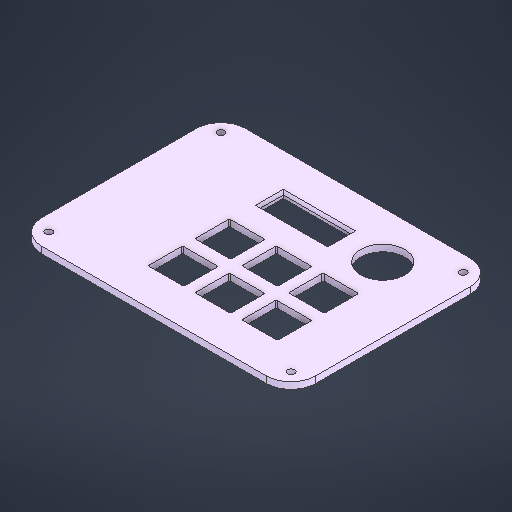
# Autodesk Inventor part: Middle
Saved by Autodesk Inventor 2026.2 (Build 302298000, 298)
## iProperties
Created: 2026-02-15
Part Number: Middle
Material: Generic
Document SubType Name: Modeling
Designer: bh
Density: 1 g/cm^3
Appearance: Default
Author: bh
Autodesk Inventor part; units mm, degrees
ref_plane "YZ Plane" through (0, 0, 0) normal (1, 0, 0) x (0, 1, 0)
ref_plane "XZ Plane" through (0, 0, 0) normal (0, 1, 0) x (-1, 0, 0)
ref_plane "XY Plane" through (0, 0, 0) normal (0, 0, 1) x (1, 0, 0)
sketch "Sketch1" plane through (0, 0, 0) normal (0, 1, 0) x (-1, 0, 0)
  line L0 (-27.2265, 26.5665) -> (-13.7265, 26.5665)
  line L1 (-27.2265, 12.5665) -> (-13.7265, 12.5665)
  line L2 (-27.7265, 26.0665) -> (-27.7265, 13.0665)
  line L3 (-13.2265, 26.0665) -> (-13.2265, 13.0665)
  arc A0 (-27.2265, 26.5665) -> (-27.7265, 26.0665) centre (-27.2265, 26.0665) ccw
  arc A1 (-13.2265, 26.0665) -> (-13.7265, 26.5665) centre (-13.7265, 26.0665) ccw
  arc A2 (-27.7265, 13.0665) -> (-27.2265, 12.5665) centre (-27.2265, 13.0665) ccw
  arc A3 (-13.7265, 12.5665) -> (-13.2265, 13.0665) centre (-13.7265, 13.0665) ccw
  line L4 (-8.1765, 26.5665) -> (4.8235, 26.5665)
  line L5 (-8.1765, 12.5665) -> (4.8235, 12.5665)
  line L6 (-8.6765, 26.0665) -> (-8.6765, 13.0665)
  arc A4 (-8.1765, 26.5665) -> (-8.6765, 26.0665) centre (-8.1765, 26.0665) ccw
  arc A5 (-8.6765, 13.0665) -> (-8.1765, 12.5665) centre (-8.1765, 13.0665) ccw
  line L7 (10.8735, 26.5665) -> (23.8735, 26.5665)
  line L8 (10.8735, 12.5665) -> (23.8735, 12.5665)
  line L9 (10.3735, 26.0665) -> (10.3735, 13.0665)
  arc A6 (10.8735, 26.5665) -> (10.3735, 26.0665) centre (10.8735, 26.0665) ccw
  arc A7 (10.3735, 13.0665) -> (10.8735, 12.5665) centre (10.8735, 13.0665) ccw
  line L10 (-28.6565, 28.2795) -> (28.4935, 28.2795)
  line L11 (-28.6565, -9.8205) -> (-28.6565, 28.2795)
  line L12 (28.4935, -9.8205) -> (28.4935, 28.2795)
  line L13 (-28.6565, 28.2795) -> (-37.9765, 28.2795)
  line L14 (-37.9765, 28.2795) -> (-37.9765, 31.2995)
  line L15 (-37.9765, 31.2995) -> (-28.6565, 31.2995)
  line L16 (-28.6565, 31.2995) -> (-28.6565, 28.2795)
  line L17 (-37.9765, 31.2995) -> (53.4235, 31.2995)
  line L18 (53.4235, 31.2995) -> (53.4235, -31.6005)
  line L19 (53.4235, -31.6005) -> (-37.9765, -31.6005)
  line L20 (-37.9765, -31.6005) -> (-37.9765, 31.2995)
  line L21 (-37.9765, -31.6005) -> (-34.6365, -31.6005)
  line L22 (-37.9765, -20.5605) -> (-37.9765, -31.6005)
  line L23 (-17.165, -31.6005) -> (-34.6365, -31.6005)
  line L24 (-37.9765, -31.6005) -> (-26.9365, -31.6005)
  line L25 (-37.9765, -16.1605) -> (-37.9765, -31.6005)
  line L26 (-14.9265, -31.6005) -> (-26.9365, -31.6005)
  line L27 (-26.9365, -31.6005) -> (-14.9265, -31.6005)
  line L28 (53.4235, -31.6005) -> (-12.9716, -31.6005)
  line L29 (53.4235, -26.4105) -> (53.4235, -31.6005)
  line L30 (-37.9765, -31.6005) -> (-2.8865, -31.6005)
  line L31 (-37.9765, -9.8205) -> (-37.9765, -31.6005)
  line L32 (63.4235, -41.6005) -> (63.4235, 41.2995)
  line L33 (63.4235, 41.2995) -> (-47.9765, 41.2995)
  line L34 (63.4235, -41.6005) -> (-47.9765, -41.6005)
  line L35 (-47.9765, -41.6005) -> (-47.9765, 41.2995)
  line L36 (-37.9008, -41.6005) -> (53.4992, -41.6005)
  line L37 (-20.9315, -41.6005) -> (-34.0815, -41.6005)
  line L38 (-47.9008, -28.4505) -> (-68.6108, -28.4505) construction
  line L39 (-37.9765, -41.6005) -> (53.4235, -41.6005)
  line L40 (-21.0072, -41.6005) -> (-34.1572, -41.6005)
  line L41 (-48.2513, 31.2983) -> (-47.9765, -31.6005)
  line L42 (-47.9903, -28.4505) -> (-68.3765, -28.4505) construction
  line L43 (-47.9765, -31.6005) -> (-37.9765, -31.6005)
  line L44 (-37.9765, -31.6005) -> (-37.9765, -41.6005)
  line L45 (-37.9765, -41.6005) -> (-47.9765, -41.6005)
  line L46 (-47.9765, -41.6005) -> (-47.9765, -31.6005)
  line L47 (-47.9765, -41.6005) -> (-27.5765, -41.6005)
  line L48 (-27.5765, -41.6005) -> (-27.5765, -9.8205)
  line L49 (-27.5765, -9.8205) -> (-47.9765, -9.8205)
  line L50 (-47.9765, -9.8205) -> (-47.9765, -41.6005)
  line L51 (-47.9765, -41.6005) -> (-15.5765, -41.6005)
  line L52 (-15.5765, -41.6005) -> (-15.5765, -9.8205)
  line L53 (-15.5765, -9.8205) -> (-47.9765, -9.8205)
  line L54 (-47.9765, -9.8205) -> (-47.9765, -41.6005)
  line L55 (-47.9765, -41.6005) -> (-9.3811, -41.6005)
  line L56 (-9.3811, -41.6005) -> (-9.3811, -28.4505)
  line L57 (-9.3811, -28.4505) -> (-47.9765, -28.4505)
  line L58 (-47.9765, -28.4505) -> (-47.9765, -41.6005)
  line L59 (-27.5765, -28.4505) -> (-15.5765, -28.4505)
  line L60 (-15.5765, -28.4505) -> (-15.5765, -16.3505)
  line L61 (-15.5765, -16.3505) -> (-27.5765, -16.3505)
  line L62 (-27.5765, -16.3505) -> (-27.5765, -28.4505)
  line L63 (-21.5765, -28.4505) -> (-21.5765, -22.4005)
  line L64 (-21.5765, -22.4005) -> (-27.5765, -22.4005)
  circle A8 centre (-21.5765, -22.4005) radius 9
  line L65 (27.5574, -41.6005) -> (-5.1303, -41.6005)
  line L66 (-5.1303, -41.6005) -> (-5.1303, -17.8005)
  line L67 (-5.1303, -17.8005) -> (27.5574, -17.8005)
  line L68 (27.5574, -17.8005) -> (27.5574, -41.6005)
  line L69 (53.4235, -22.9498) -> (23.0635, -22.9498)
  line L70 (23.0635, -22.9498) -> (-3.5365, -22.9498)
  line L71 (23.0635, -17.8005) -> (23.0635, -26.6005)
  line L72 (23.0635, -26.6005) -> (-3.7865, -26.6005)
  line L73 (-3.7865, -26.6005) -> (-3.7865, -17.8005)
  line L74 (-3.7865, -17.8005) -> (23.0635, -17.8005)
  line L75 (23.0635, -17.8005) -> (23.0635, -26.6005)
  line L76 (-4.0365, -26.8505) -> (23.3135, -26.8505)
  line L77 (23.3135, -26.8505) -> (23.3135, -17.5505)
  line L78 (23.3135, -17.5505) -> (-4.0365, -17.5505)
  line L79 (-4.0365, -17.5505) -> (-4.0365, -26.8505)
  line L80 (-48.1765, 14.1732) -> (-27.9265, 14.1732)
  line L81 (-27.7265, 13.0665) -> (-27.7265, 13.0665)
  line L82 (-20.7265, 12.5665) -> (-20.7265, 12.5665)
  line L83 (-20.7265, 12.5665) -> (-20.7265, 12.5665)
  line L84 (-27.7265, 13.0665) -> (-27.7265, 13.0665)
  line L85 (-27.7265, 19.5665) -> (-13.2265, 19.5665)
  line L86 (-13.2265, 13.0665) -> (-13.2265, 13.0665)
  line L87 (-8.1765, 12.5665) -> (5.3235, 12.5665)
  arc A9 (-8.6765, 13.0665) -> (-8.1765, 12.5665) centre (-8.1765, 13.0665) ccw
  arc A10 (5.3235, 12.5665) -> (5.8235, 13.0665) centre (5.3235, 13.0665) ccw
  line L88 (-8.6765, 26.0665) -> (-8.6765, 13.0665)
  line L89 (5.8235, 26.0665) -> (5.8235, 13.0665)
  line L90 (-8.1765, 26.5665) -> (5.3235, 26.5665)
  arc A11 (-8.1765, 26.5665) -> (-8.6765, 26.0665) centre (-8.1765, 26.0665) ccw
  arc A12 (5.8235, 26.0665) -> (5.3235, 26.5665) centre (5.3235, 26.0665) ccw
  line L91 (10.8735, 12.5665) -> (24.3735, 12.5665)
  arc A13 (10.3735, 13.0665) -> (10.8735, 12.5665) centre (10.8735, 13.0665) ccw
  arc A14 (24.3735, 12.5665) -> (24.8735, 13.0665) centre (24.3735, 13.0665) ccw
  line L92 (10.3735, 26.0665) -> (10.3735, 13.0665)
  line L93 (24.8735, 26.0665) -> (24.8735, 13.0665)
  line L94 (10.8735, 26.5665) -> (24.3735, 26.5665)
  arc A15 (10.8735, 26.5665) -> (10.3735, 26.0665) centre (10.8735, 26.0665) ccw
  arc A16 (24.8735, 26.0665) -> (24.3735, 26.5665) centre (24.3735, 26.0665) ccw
  line L95 (17.3735, 12.5665) -> (17.3735, 12.5665)
  line L96 (17.3735, 12.5665) -> (17.3735, 12.5665)
  line L97 (24.8735, 13.0665) -> (24.8735, 13.0665)
  line L98 (-28.6565, 7.0165) -> (-28.6565, 9.2295)
  line L99 (-28.6565, 9.2295) -> (-27.2265, 9.2295)
  line L100 (-27.2265, -6.4831) -> (-13.7265, -6.4831)
  arc A17 (-27.7265, -5.9831) -> (-27.2265, -6.4831) centre (-27.2265, -5.9831) ccw
  arc A18 (-13.7265, -6.4831) -> (-13.2265, -5.9831) centre (-13.7265, -5.9831) ccw
  line L101 (-27.7265, 7.0169) -> (-27.7265, -5.9831)
  line L102 (-13.2265, 7.0169) -> (-13.2265, -5.9831)
  line L103 (-27.2265, 7.5169) -> (-13.7265, 7.5169)
  arc A19 (-27.2265, 7.5169) -> (-27.7265, 7.0169) centre (-27.2265, 7.0169) ccw
  arc A20 (-13.2265, 7.0169) -> (-13.7265, 7.5169) centre (-13.7265, 7.0169) ccw
  line L104 (-8.6765, 7.0169) -> (-8.6765, -5.9831)
  arc A21 (-8.1765, 7.5169) -> (-8.6765, 7.0169) centre (-8.1765, 7.0169) ccw
  line L105 (-8.1765, -6.4831) -> (4.8235, -6.4831)
  arc A22 (-8.6765, -5.9831) -> (-8.1765, -6.4831) centre (-8.1765, -5.9831) ccw
  line L106 (-8.1765, 7.5169) -> (4.8235, 7.5169)
  line L107 (10.3735, 7.0169) -> (10.3735, -5.9831)
  line L108 (10.8735, 7.5169) -> (23.8735, 7.5169)
  arc A23 (10.8735, 7.5169) -> (10.3735, 7.0169) centre (10.8735, 7.0169) ccw
  line L109 (10.8735, -6.4831) -> (23.8735, -6.4831)
  arc A24 (10.3735, -5.9831) -> (10.8735, -6.4831) centre (10.8735, -5.9831) ccw
  line L110 (-27.7265, -5.9831) -> (-27.7265, -5.9831)
  line L111 (-20.7265, -6.4831) -> (-20.7265, -6.4831)
  line L112 (-20.7265, -6.4831) -> (-20.7265, -6.4831)
  line L113 (-27.7265, -5.9831) -> (-27.7265, -5.9831)
  line L114 (-13.2265, -5.9831) -> (-13.2265, -5.9831)
  line L115 (-8.6765, 7.0169) -> (-8.6765, -5.9831)
  arc A25 (-8.1765, 7.5169) -> (-8.6765, 7.0169) centre (-8.1765, 7.0169) ccw
  line L116 (5.8235, 7.0169) -> (5.8235, -5.9831)
  line L117 (-8.1765, 7.5169) -> (5.3235, 7.5169)
  arc A26 (5.8235, 7.0169) -> (5.3235, 7.5169) centre (5.3235, 7.0169) ccw
  line L118 (-8.1765, -6.4831) -> (5.3235, -6.4831)
  arc A27 (5.3235, -6.4831) -> (5.8235, -5.9831) centre (5.3235, -5.9831) ccw
  arc A28 (-8.6765, -5.9831) -> (-8.1765, -6.4831) centre (-8.1765, -5.9831) ccw
  arc A29 (10.3735, -5.9831) -> (10.8735, -6.4831) centre (10.8735, -5.9831) ccw
  line L119 (10.8735, -6.4831) -> (24.3735, -6.4831)
  arc A30 (24.3735, -6.4831) -> (24.8735, -5.9831) centre (24.3735, -5.9831) ccw
  arc A31 (24.8735, 7.0169) -> (24.3735, 7.5169) centre (24.3735, 7.0169) ccw
  line L120 (24.8735, 7.0169) -> (24.8735, -5.9831)
  line L121 (10.8735, 7.5169) -> (24.3735, 7.5169)
  arc A32 (10.8735, 7.5169) -> (10.3735, 7.0169) centre (10.8735, 7.0169) ccw
  line L122 (17.3735, -6.4831) -> (17.3735, -6.4831)
  line L123 (17.3735, -6.4831) -> (17.3735, -6.4831)
  line L124 (24.8735, -5.9831) -> (24.8735, -5.9831)
  line L125 (10.3735, 7.0169) -> (10.3735, -5.9831)
  line L126 (-27.7265, 7.0169) -> (-27.7265, -5.9831)
  arc A33 (-27.2265, 7.5169) -> (-27.7265, 7.0169) centre (-27.2265, 7.0169) ccw
  line L127 (-27.2265, -6.4831) -> (-14.2265, -6.4831)
  arc A34 (-27.7265, -5.9831) -> (-27.2265, -6.4831) centre (-27.2265, -5.9831) ccw
  line L128 (-27.2265, 7.5169) -> (-14.2265, 7.5169)
  line L129 (-27.7265, 7.0169) -> (-27.7265, -5.9831)
  arc A35 (-27.2265, 7.5169) -> (-27.7265, 7.0169) centre (-27.2265, 7.0169) ccw
  line L130 (-13.2265, 7.0169) -> (-13.2265, -5.9831)
  line L131 (-27.2265, 7.5169) -> (-13.7265, 7.5169)
  arc A36 (-13.2265, 7.0169) -> (-13.7265, 7.5169) centre (-13.7265, 7.0169) ccw
  line L132 (-27.2265, -6.4831) -> (-13.7265, -6.4831)
  arc A37 (-13.7265, -6.4831) -> (-13.2265, -5.9831) centre (-13.7265, -5.9831) ccw
  arc A38 (-27.7265, -5.9831) -> (-27.2265, -6.4831) centre (-27.2265, -5.9831) ccw
  point P0 (10.8735, 26.5665)
  point P1 (10.8735, 12.5665)
  point P2 (10.3735, 13.0665)
  point P3 (-8.1765, 12.5665)
  point P4 (-8.6765, 13.0665)
  point P5 (-8.6765, 26.0665)
  point P6 (-14.2265, 26.5665)
  point P7 (-13.2265, 13.0665)
  point P8 (-14.2265, 12.5665)
  point P9 (-2.8865, -17.0492)
  point P10 (-6.5815, -26.4105)
  point P11 (23.7135, -17.6392)
  point P12 (23.3135, -17.8005)
  point P13 (-4.0365, -17.8005)
  point P14 (-1.6765, 12.5665)
  point P15 (-8.6765, 19.5665)
  point P16 (-8.6765, 0.5169)
  point P17 (-1.6765, -6.4831)
  point P18 (-8.1765, 7.5169)
  point P19 (-27.2265, 7.5169)
  point P20 (24.8735, 7.0169)
  point P21 (10.8735, 7.5169)
  point P22 (24.8735, 13.0665)
  point P23 (24.8735, 26.0665)
  point P24 (-20.7265, -6.4831)
  dimension "d8" = 9.32
  dimension "d9" = 3.02
  dimension "d11" = 62.9
  dimension "d24" = 10
  dimension "d25" = 10
  dimension "d26" = 10
  dimension "d63" = 20.4
  dimension "d65" = 13.15
  dimension "d66" = 12.1
  dimension "d67" = 18
  dimension "d68" = 23.8
  dimension "d69" = 30.36
  dimension "d70" = 26.6
  dimension "d71" = 8.8
  dimension "d72" = 0.25
  dimension "d75" = 20.25
  dimension "d76" = 0
  dimension "d77" = 0
  dimension "d78" = 14.5
  dimension "d79" = 0
  dimension "d80" = 0
  constraints: 266 end point, 76 point on circle, 39 centre point, 24 horizontal, 23 parallel, 22 point on line, 12 perpendicular, 9 vertical, 6 midpoint, 1 coincident, 3 other
  measures "d8" distance of L14.end L15.end
  measures "d9" distance of L13.end L14.end
  measures "d11" distance of L17.end L18.end
  measures "d24" distance between parallel lines of L18 L32
  measures "d25" distance between parallel lines of L19 L34
  measures "d26" distance between parallel lines of L20 L35
  measures "d63" distance of L49.end L48.end
  measures "d65" distance of L56.end L55.end
  measures "d66" distance of L60.end L59.end
  measures "d67" diameter of A8
  measures "d68" distance of L65.end L66.end
  measures "d69" distance of L69.start L69.end
  measures "d70" distance of L69.end L70.end
  measures "d71" distance of L71.start L71.end
  measures "d72" distance between parallel lines of L72 L76
  measures "d75" distance of L80.start L80.end
  measures "d76" distance of L82.start L82.end
  measures "d77" distance of L82.end L83.end
  measures "d78" distance of L85.start L85.end
  measures "d79" distance of L95.start L95.end
  measures "d80" distance of L95.end L96.end
extrude "Extrusion1" add sketch "Sketch1" along normal blind 2.7 contours L49 L20 L80 L11 | L11 L16 L17 L18 L69 L68 L67 L77 L78 L79 L66 L19 L56 L57 A8 L52 L53 L49 | L49 L48 A8 L57 L20 | L53 L52 A8 L48 | L49 L35 L80 L20 | L20 L57 L35 L49 | L80 L35 L33 L32 L34 L68 L19 L18 L17 L15 L14 L20 | L20 L13 L11 L80 | A8 L48 L19 L20 L57 | L14 L15 L16 L13 | L57 L20 L43 L35 | A8 L52 L19 L48 | L43 L44 L34 L35 | L57 L56 L19 L52 A8 | L19 L48 L34 L44 | L19 L52 L34 L48 | L19 L56 L34 L52 | L18 L19 L68 L69 | L19 L66 L34 L56 | L69 L77 L67 L68 | L68 L19 L66 L67 L79 L76 L77 L69 | L19 L68 L34 L66 | A17 L101 A19 L103 A20 L102 A18 L100
fillet "Fillet1" radius 10 4 edges at (47.9765, 1.35, -41.6005) (47.9765, 1.35, 41.2995) (-63.4235, 1.35, 41.2995) (-63.4235, 1.35, -41.6005)
sketch "Sketch4" plane through (0, 0, 0) normal (0, -1, 0) x (1, 0, 0)
  line L0 (37.9765, -41.6005) -> (-53.4235, -41.6005) projected
  line L1 (47.9765, 31.2995) -> (47.9765, -31.6005) projected
  line L2 (-53.4235, 41.2995) -> (37.9765, 41.2995) projected
  line L3 (-63.4235, -31.6005) -> (-63.4235, 31.2995) projected
  line L4 (45.0476, -38.6715) -> (41.512, -35.136)
  line L5 (45.0476, -38.6715) -> (50.0476, -38.6715) construction
  line L6 (-60.4946, 38.3706) -> (-56.959, 34.8351)
  line L7 (45.0476, 38.3706) -> (41.512, 34.8351)
  line L8 (-60.4946, -38.6715) -> (-56.959, -35.136)
  circle A0 centre (41.512, -35.136) radius 1.45
  circle A1 centre (-56.959, -35.136) radius 1.45
  circle A2 centre (-56.959, 34.8351) radius 1.45
  circle A3 centre (41.512, 34.8351) radius 1.45
  arc A4 (-63.4235, -31.6005) -> (-53.4235, -41.6005) centre (-53.4235, -31.6005) ccw projected
  arc A5 (37.9765, -41.6005) -> (47.9765, -31.6005) centre (37.9765, -31.6005) ccw projected
  arc A6 (47.9765, 31.2995) -> (37.9765, 41.2995) centre (37.9765, 31.2995) ccw projected
  arc A7 (-53.4235, 41.2995) -> (-63.4235, 31.2995) centre (-53.4235, 31.2995) ccw projected
  point P0 (0, 0)
  dimension "d28" = 5
  dimension "d29" = 135
  dimension "d31" = 5
  dimension "d32" = 5
  dimension "d33" = 5
  dimension "d34" = 2.9
  dimension "d35" = 2.9
  dimension "d36" = 2.9
  dimension "d37" = 2.9
  constraints: 10 end point, 4 centre point, 4 coincident, 1 equal length, 1 horizontal
  measures "d28" distance of L4.start L4.end
  measures "d29" angle of L5 L4
  measures "d31" distance of L6.start L6.end
  measures "d32" distance of L7.start L7.end
  measures "d33" distance of L8.start L8.end
  measures "d34" diameter of A0
  measures "d35" diameter of A1
  measures "d36" diameter of A2
  measures "d37" diameter of A3
extrude "Extrusion3" cut sketch "Sketch4" against normal blind 3 contours A0 | A1 | A2 | A3
chamfer "Chamfer1" distance 1 angle 45 4 edges at (-9.6385, 2.7, -17.5505) (-23.3135, 2.7, -22.2005) (-9.6385, 2.7, -26.8505) (4.0365, 2.7, -22.2005)
sketch "Sketch5" plane through (0, 0, 0) normal (0, -1, 0) x (1, 0, 0)
  line L0 (11.1455, -33.7067) -> (-37.5786, -33.7067)
  line L1 (-37.5786, -33.7067) -> (-37.5786, -13.6492)
  line L2 (-37.5786, -13.6492) -> (11.1455, -13.6492)
  line L3 (11.1455, -13.6492) -> (11.1455, -33.7067)
  point P0 (0, 0)
  constraints: 8 end point, 2 parallel, 1 horizontal, 1 perpendicular
extrude "Extrusion4" cut sketch "Sketch5" against normal blind 0.5
extrude "Extrusion5" cut sketch "Sketch1" along normal blind 2.7 contours A17 L101 A19 L103 A20 L102 A18 L100 | A21 L106 L117 A26 L116 A27 L118 L105 A22 L104
body "Solid1"
